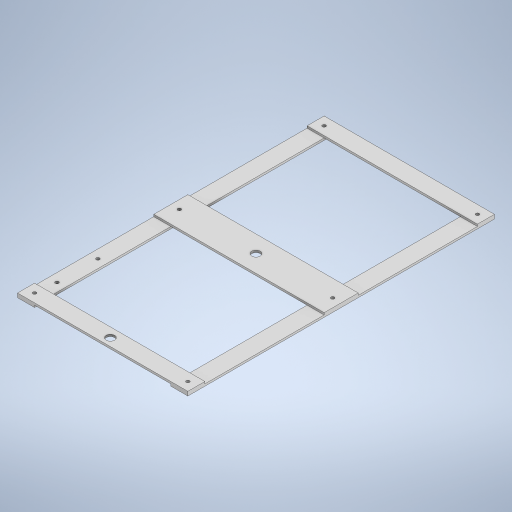
# Autodesk Inventor part: Base Platform
Saved by Autodesk Inventor 2024 (Build 280153000, 153)
## iProperties
Created: 2024-02-05
Part Number: Base Platform
Material: Generic
Document SubType Name: Modeling
Designer: Ramji Yadav
Density: 1 g/cm^3
Appearance: Default
Author: Ramji Yadav
Autodesk Inventor part; units mm, degrees
ref_plane "YZ Plane" through (0, 0, 0) normal (1, 0, 0) x (0, 1, 0)
ref_plane "XZ Plane" through (0, 0, 0) normal (0, 1, 0) x (-1, 0, 0)
ref_plane "XY Plane" through (0, 0, 0) normal (0, 0, 1) x (1, 0, 0)
sketch "Sketch1" plane through (0, 0, 0) normal (0, 0, 1) x (1, 0, 0)
  line L0 (0, 0) -> (25, 0)
  line L1 (25, 0) -> (25, 3)
  line L2 (25, 3) -> (0, 3)
  line L3 (0, 3) -> (0, 0)
  dimension "d0" = 25
  dimension "d1" = 3
  constraints: 8 end point, 2 parallel, 1 horizontal, 1 perpendicular
  measures "d0" distance of L2.end L1.end
  measures "d1" distance of L1.end L0.end
extrude "Extrusion1" add sketch "Sketch1" along normal blind 450
sketch "Sketch2" plane through (0, 3, 0) normal (0, 1, 0) x (1, 0, 0)
  line L0 (0, 0) -> (0, -450) projected
  line L1 (0, 0) -> (250, 0)
  line L2 (250, 0) -> (250, -25)
  line L3 (250, -25) -> (0, -25)
  line L4 (0, -25) -> (0, 0)
  dimension "d4" = 250
  dimension "d5" = 25
  constraints: 8 end point, 2 parallel, 1 horizontal, 1 perpendicular
  measures "d4" distance of L2.end L3.end
  measures "d5" distance of L1.end L2.end
extrude "Extrusion2" add sketch "Sketch2" along normal blind 3
sketch "Sketch3" plane through (0, 3, 450) normal (0, 1, 0) x (1, 0, 0)
  line L0 (0, 450) -> (0, 0) projected
  line L1 (0, 0) -> (250, 0)
  line L2 (250, 0) -> (250, 25)
  line L3 (250, 25) -> (0, 25)
  line L4 (0, 25) -> (0, 0)
  dimension "d8" = 250
  dimension "d9" = 25
  constraints: 8 end point, 2 parallel, 1 horizontal, 1 perpendicular
  measures "d8" distance of L3.end L2.end
  measures "d9" distance of L2.end L1.end
extrude "Extrusion3" add sketch "Sketch3" along normal blind 3
sketch "Sketch4" plane through (0, 3, 0) normal (0, -1, 0) x (1, 0, 0)
  line L0 (250, 0) -> (0, 0) projected
  line L1 (250, 0) -> (225, 0)
  line L2 (225, 0) -> (225, 450)
  line L3 (225, 450) -> (250, 450)
  line L4 (250, 450) -> (250, 0)
  dimension "d12" = 25
  dimension "d13" = 450
  constraints: 8 end point, 2 parallel, 1 horizontal, 1 perpendicular
  measures "d12" distance of L2.end L3.end
  measures "d13" distance of L1.end L2.end
extrude "Extrusion4" add sketch "Sketch4" along normal blind 3
sketch "Sketch5" plane through (0, 3, 25) normal (0, 1, 0) x (1, 0, 0)
  line L0 (0, 25) -> (0, -175)
  line L1 (0, 0) -> (0, -400) projected
  line L2 (0, -175) -> (250, -175)
  line L3 (250, -175) -> (250, -225)
  line L4 (250, -225) -> (0, -225)
  line L5 (0, -225) -> (0, -175)
  dimension "d16" = 200
  dimension "d17" = 250
  dimension "d18" = 50
  constraints: 10 end point, 2 parallel, 1 horizontal, 1 perpendicular, 1 point on line
  measures "d16" distance of L0.start L0.end
  measures "d17" distance of L3.end L4.end
  measures "d18" distance of L2.end L3.end
extrude "Extrusion5" add sketch "Sketch5" along normal blind 3
sketch "Sketch6" plane through (0, 6, 0) normal (0, 1, 0) x (1, 0, 0)
  line L0 (25, -25) -> (0, -25) projected
  line L1 (0, 0) -> (0, -25) projected
  line L2 (25, -25) -> (0, -25)
  line L3 (0, -25) -> (0, 0)
  line L4 (0, 0) -> (25, 0)
  line L5 (25, 0) -> (25, -25)
  line L6 (25, -25) -> (0, 0)
  line L7 (225, 0) -> (25, 0) projected
  line L8 (25, 0) -> (0, -25)
  circle A0 centre (12.5, -12.5) radius 2.5
  line L9 (0, -450) -> (250, -450) projected
  line L10 (250, -425) -> (0, -425) projected
  line L11 (0, -450) -> (25, -450)
  line L12 (25, -450) -> (25, -425)
  line L13 (25, -425) -> (0, -425)
  line L14 (0, -425) -> (0, -450)
  line L15 (250, -450) -> (225, -450)
  line L16 (225, -450) -> (225, -425)
  line L17 (225, -425) -> (250, -425)
  line L18 (250, -425) -> (250, -450)
  line L19 (0, -450) -> (25, -425)
  line L20 (25, -450) -> (0, -425)
  line L21 (250, -450) -> (225, -425)
  line L22 (225, -425) -> (225, -250) projected
  line L23 (225, -450) -> (250, -425)
  circle A1 centre (237.5, -437.5) radius 2.5
  circle A2 centre (12.5, -437.5) radius 2.5
  line L24 (250, -25) -> (250, 0) projected
  line L25 (225, -25) -> (250, -25) projected
  line L26 (250, 0) -> (225, 0)
  line L27 (225, 0) -> (225, -25)
  line L28 (225, -25) -> (250, -25)
  line L29 (250, -25) -> (250, 0)
  line L30 (250, -25) -> (225, 0)
  line L31 (225, 0) -> (225, -25) projected
  line L32 (225, 0) -> (225, -25)
  line L33 (225, -25) -> (250, 0)
  circle A3 centre (237.5, -12.5) radius 2.5
  dimension "d21" = 5
  dimension "d22" = 5
  dimension "d23" = 5
  dimension "d24" = 5
  constraints: 50 end point, 9 equal length, 6 perpendicular, 4 centre point, 4 horizontal, 4 midpoint, 4 point on line
  measures "d21" diameter of A0
  measures "d22" diameter of A1
  measures "d23" diameter of A2
  measures "d24" diameter of A3
extrude "Extrusion6" cut sketch "Sketch6" against normal blind 100 contours A0 L8 L6 | L6 L8 A0 | A0 L6 L8 | L8 L6 A0 | A3 L33 L30 | L30 L33 A3 | A3 L30 L33 | L33 L30 A3 | A2 L20 L19 | L19 L20 A2 | L20 L19 A2 | A2 L19 L20 | A1 L21 L23 | L23 L21 A1 | L21 L23 A1 | A1 L23 L21
sketch "Sketch7" plane through (0, 6, 25) normal (0, 1, 0) x (1, 0, 0)
  circle A0 centre (12.5, -200) radius 2.5
  line L0 (0, -175) -> (0, -225) projected
  line L1 (0, -225) -> (250, -225) projected
  circle A1 centre (237.5, -200) radius 2.5
  line L2 (250, -225) -> (250, -175) projected
  line L3 (250, -175) -> (0, -175) projected
  point P0 (0, 25)
  dimension "d27" = 5
  dimension "d28" = 12.5
  dimension "d29" = 25
  dimension "d30" = 5
  dimension "d31" = 12.5
  dimension "d32" = 25
  constraints: 2 centre point
  measures "d27" diameter of A0
  measures "d28" distance from line of L0 A0.centre
  measures "d29" distance from line of L1 A0.centre
  measures "d30" diameter of A1
  measures "d31" distance from line of L2 A1.centre
  measures "d32" distance from line of L3 A1.centre
extrude "Extrusion7" cut sketch "Sketch7" against normal blind 100 contours A0 | A1
thread "Thread1" size "M5x0.8" class "6H" standard "ANSI Metric M Profile" full length
thread "Thread2" size "M5x0.8" class "6H" standard "ANSI Metric M Profile" full length
thread "Thread3" size "M5x0.8" class "6H" standard "ANSI Metric M Profile" full length
thread "Thread4" size "M5x0.8" class "6H" standard "ANSI Metric M Profile" full length
thread "Thread5" size "M5x0.8" class "6H" standard "ANSI Metric M Profile" full length
thread "Thread6" size "M5x0.8" class "6H" standard "ANSI Metric M Profile" full length
sketch "Sketch8" plane through (0, 6, 25) normal (0, 1, 0) x (1, 0, 0)
  circle A0 centre (12.5, -200) radius 2.5 projected
  circle A1 centre (237.5, -200) radius 2.5 projected
  circle A2 centre (125, -200) radius 6.35
  line L0 (250, -225) -> (250, -175) projected
  point P0 (0, 25)
  dimension "d47" = 12.7
  dimension "d48" = 125
  constraints: 1 centre point
  measures "d47" diameter of A2
  measures "d48" distance from line of L0 A2.centre
extrude "Extrusion8" cut sketch "Sketch8" against normal blind 10 contours A2
sketch "Sketch9" plane through (0, 6, 450) normal (0, 1, 0) x (1, 0, 0)
  circle A0 centre (125, 11.2801) radius 6.35
  line L0 (250, 0) -> (250, 25) projected
  point P0 (0, 450)
  dimension "d51" = 12.7
  dimension "d52" = 125
  constraints: 1 centre point
  measures "d51" diameter of A0
  measures "d52" distance from line of L0 A0.centre
extrude "Extrusion9" cut sketch "Sketch9" against normal through all
thread "Thread7" size "M14x2" class "6H" standard "ANSI Metric M Profile" full length
sketch "Sketch10" plane through (0, 3, 425) normal (0, 1, 0) x (1, 0, 0)
  line L0 (25, 425) -> (25, -25) projected
  line L1 (0, 425) -> (0, -25) projected
  line L2 (25, 0.3749) -> (0, 0.3749)
  line L3 (0, 0.3749) -> (0, 100.3749)
  line L4 (0, 100.3749) -> (25, 100.3749)
  line L5 (25, 100.3749) -> (25, 0.3749)
  circle A0 centre (12.5, 20.3749) radius 2.5
  circle A1 centre (12.5, 80.3749) radius 2.5
  point P0 (12.5, 0.3749)
  point P1 (12.5, 100.3749)
  dimension "d57" = 100
  dimension "d58" = 5
  dimension "d59" = 5
  dimension "d60" = 20
  dimension "d61" = 20
  dimension "d62" = 12.5
  dimension "d63" = 12.5
  constraints: 8 end point, 2 centre point, 2 midpoint, 2 parallel, 2 point on line, 1 horizontal, 1 perpendicular
  measures "d57" distance of L2.end L3.end
  measures "d58" diameter of A0
  measures "d59" diameter of A1
  measures "d60" distance of point (12.5, 0.375) A0.centre
  measures "d61" distance of A1.centre point (12.5, 100.375)
  measures "d62" distance from line of L1 A0.centre
  measures "d63" distance from line of L1 A1.centre
extrude "Extrusion10" cut sketch "Sketch10" against normal blind 10 contours A0 | A1
thread "Thread8" size "M5x0.8" class "6H" standard "ANSI Metric M Profile" full length
thread "Thread9" size "M5x0.8" class "6H" standard "ANSI Metric M Profile" full length
body "Solid1"
